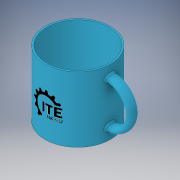
# Autodesk Inventor part: 練習二
Saved by Autodesk Inventor 2017 (Build 210142000, 142)
## iProperties
Part Number: 練習二
Material: 一般
Document SubType Name: Modeling
Designer: user
Density: 1 g/cm^3
Appearance: 青綠色
Author: user
Autodesk Inventor part; units mm, degrees
ref_plane "YZ Plane" through (0, 0, 0) normal (1, 0, 0) x (0, 1, 0)
sketch "草圖1" plane through (0, 0, 0) normal (0, 1, 0) x (-1, 0, 0)
  circle A0 centre (0, 0) radius 40
  dimension "d0" = 80
  constraints: 1 centre point, 1 coincident
  measures "d0" diameter of A0
extrude "擠出1" add sketch "草圖1" along normal blind 80
shell "薄殼3" thickness 2 removed faces 1 at (12.1058, 80, -2.3153)
sketch "草圖6" plane through (0, 0, 0) normal (0, 0, 1) x (1, 0, 0)
  line L0 (40, 0) -> (40, 80) projected
  arc A0 (38, 14.077) -> (38, 65.923) centre (40, 40) ccw
  line L1 (-40, 0) -> (40, 0) projected
  line L2 (38, 2) -> (38, 80) construction
  point P0 (0, 0)
  dimension "d23" = 52
  dimension "d24" = 40
  constraints: 2 point on circle, 2 point on line, 1 centre point, 1 midpoint
  measures "d23" diameter of A0
  measures "d24" distance from line of A0.centre L1
ref_plane "工作平面2" through (38, 65.923, 0) normal (-0.997, -0.0769, 0) x (0.0769, -0.997, 0)
sketch "草圖7" plane through (38, 65.923, 0) normal (-0.997, -0.0769, 0) x (0.0769, -0.997, 0)
  ellipse E0 centre (0, 0) end of major axis (0, -6) minor radius 4
  point P0 (62.8046, 0)
  dimension "d25" = 4
  dimension "d26" = 6
  constraints: 2 other
sweep "掃掠3" add profiles "草圖7" path "草圖6" path curves A0
fillet "圓角5" radius 2 2 edges at (39.5474, 66.0021, 6) (39.5474, 13.9979, 6)
ref_plane "工作平面3" through (0, 0, 70) normal (0, 0, 1) x (1, 0, 0)
sketch "草圖11" plane through (0, 0, 70) normal (0, 0, 1) x (1, 0, 0)
  line L0 (-18.4453, 56.0809) -> (19.5727, 56.0809)
  line L1 (19.5727, 56.0809) -> (19.5727, 18.0629)
  line L2 (19.5727, 18.0629) -> (-18.4453, 18.0629)
  line L3 (-18.4453, 18.0629) -> (-18.4453, 56.0809)
  point P0 (0, 0)
  constraints: 2 other
decal "印花2"
